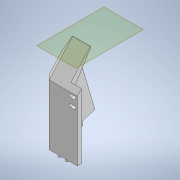
# Autodesk Inventor part: blotnik_v3_part_1
Saved by Autodesk Inventor 2022.3 (Build 263350000, 350)
## iProperties
Created: 2022-10-25
Part Number: blotnik_v3_part_1
Material: Generic
Document SubType Name: Modeling
Designer: Kamil
Density: 1 g/cm^3
Appearance: Default
Author: Kamil
Autodesk Inventor part; units mm, degrees
(part 1 of 2)
ref_plane "YZ Plane" through (0, 0, 0) normal (1, 0, 0) x (0, 1, 0)
ref_plane "XZ Plane" through (0, 0, 0) normal (0, 1, 0) x (-1, 0, 0)
sketch "Sketch1" plane through (0, 0, 0) normal (1, 0, 0) x (0, 1, 0)
  line L0 (-91.9132, 90.5719) -> (-91.9132, 0.5719)
  line L1 (-91.9132, 0.5719) -> (48.2351, 0.5719)
  arc A0 (48.2351, 0.5719) -> (67.9385, 0.5719) centre (58.0868, 2.2876) ccw
  line L2 (67.9385, 0.5719) -> (198.2351, 0.5719)
  arc A1 (198.2351, 0.5719) -> (217.9385, 0.5719) centre (208.0868, 2.2876) ccw
  line L3 (217.9385, 0.5719) -> (338.2351, 0.5719)
  arc A2 (338.2351, 0.5719) -> (357.9385, 0.5719) centre (348.0868, 2.2876) ccw
  line L4 (357.9385, 0.5719) -> (387.824, 0.5719)
  arc A3 (387.824, 0.5719) -> (392.824, 1.9116) centre (387.824, 10.5719) ccw
  line L5 (392.824, 1.9116) -> (465.5868, 43.9213)
  arc A4 (465.5868, 43.9213) -> (453.0868, 90.5719) centre (453.0868, 65.5719) ccw
  line L6 (453.0868, 90.5719) -> (215.5868, 90.5719)
  arc A5 (215.5868, 90.5719) -> (200.5868, 90.5719) centre (208.0868, 90.5719) ccw
  line L7 (200.5868, 90.5719) -> (65.5868, 90.5719)
  arc A6 (65.5868, 90.5719) -> (50.5868, 90.5719) centre (58.0868, 90.5719) ccw
  line L8 (50.5868, 90.5719) -> (-91.9132, 90.5719)
  line L9 (394.4234, 30.0809) -> (384.8369, 44.4607)
  arc A7 (384.8369, 46.6796) -> (384.8369, 44.4607) centre (386.501, 45.5701) ccw
  line L10 (384.8369, 46.6796) -> (394.4264, 61.0622)
  arc A8 (398.0904, 59.9525) -> (394.4264, 61.0622) centre (396.0904, 59.9527) ccw
  line L11 (398.0904, 59.9525) -> (398.0875, 31.1901)
  arc A9 (394.4234, 30.0809) -> (398.0875, 31.1901) centre (396.0875, 31.1903) ccw
  line L12 (46.0868, 47.6815) -> (11.9586, 47.6815)
  arc A10 (11.0641, 51.4704) -> (11.9586, 47.6815) centre (11.9586, 49.6815) ccw
  line L13 (11.0641, 51.4704) -> (45.1924, 68.5345)
  arc A11 (48.0868, 66.7457) -> (45.1924, 68.5345) centre (46.0868, 66.7457) ccw
  line L14 (48.0868, 66.7457) -> (48.0868, 49.6815)
  arc A12 (46.0868, 47.6815) -> (48.0868, 49.6815) centre (46.0868, 49.6815) ccw
  line L15 (278.9812, 39.5345) -> (319.3287, 19.3608)
  arc A13 (318.4343, 15.5719) -> (319.3287, 19.3608) centre (318.4343, 17.5719) ccw
  line L16 (318.4343, 15.5719) -> (237.7393, 15.5719)
  arc A14 (236.8448, 19.3608) -> (237.7393, 15.5719) centre (237.7393, 17.5719) ccw
  line L17 (236.8448, 19.3608) -> (277.1924, 39.5345)
  arc A15 (278.9812, 39.5345) -> (277.1924, 39.5345) centre (278.0868, 37.7457) ccw
  line L18 (367.8331, 75.5719) -> (388.3444, 75.5719)
  arc A16 (390.0084, 72.4624) -> (388.3444, 75.5719) centre (388.3444, 73.5719) ccw
  line L19 (390.0084, 72.4624) -> (379.7522, 57.0798)
  arc A17 (376.4241, 57.0798) -> (379.7522, 57.0798) centre (378.0882, 58.1892) ccw
  line L20 (376.4241, 57.0798) -> (366.169, 72.4625)
  arc A18 (367.8331, 75.5719) -> (366.169, 72.4625) centre (367.8331, 73.5719) ccw
  line L21 (361.7509, 61.0619) -> (371.3389, 46.6799)
  arc A19 (371.3388, 44.461) -> (371.3389, 46.6799) centre (369.6748, 45.5705) ccw
  line L22 (371.3388, 44.461) -> (361.7508, 30.0806)
  arc A20 (358.0868, 31.1901) -> (361.7508, 30.0806) centre (360.0868, 31.1901) ccw
  line L23 (358.0868, 31.1901) -> (358.0868, 59.9525)
  arc A21 (361.7509, 61.0619) -> (358.0868, 59.9525) centre (360.0868, 59.9525) ccw
  line L24 (89.1243, 75.5719) -> (177.0493, 75.5719)
  arc A22 (177.8875, 71.756) -> (177.0493, 75.5719) centre (177.0493, 73.5719) ccw
  line L25 (177.8875, 71.756) -> (133.9249, 51.4656)
  arc A23 (132.2487, 51.4656) -> (133.9249, 51.4656) centre (133.0868, 53.2815) ccw
  line L26 (132.2487, 51.4656) -> (88.2861, 71.756)
  arc A24 (89.1243, 75.5719) -> (88.2861, 71.756) centre (89.1243, 73.5719) ccw
  line L27 (-11.0188, 39.5345) -> (29.3287, 19.3608)
  arc A25 (28.4343, 15.5719) -> (29.3287, 19.3608) centre (28.4343, 17.5719) ccw
  line L28 (28.4343, 15.5719) -> (-52.2607, 15.5719)
  arc A26 (-53.1552, 19.3608) -> (-52.2607, 15.5719) centre (-52.2607, 17.5719) ccw
  line L29 (-53.1552, 19.3608) -> (-12.8076, 39.5345)
  arc A27 (-11.0188, 39.5345) -> (-12.8076, 39.5345) centre (-11.9132, 37.7457) ccw
  line L30 (117.2208, 43.756) -> (70.9249, 22.3887)
  arc A28 (68.0868, 24.2046) -> (70.9249, 22.3887) centre (70.0868, 24.2046) ccw
  line L31 (68.0868, 24.2046) -> (68.0868, 66.9392)
  arc A29 (70.9249, 68.7551) -> (68.0868, 66.9392) centre (70.0868, 66.9392) ccw
  line L32 (70.9249, 68.7551) -> (117.2208, 47.3878)
  arc A30 (117.2208, 43.756) -> (117.2208, 47.3878) centre (116.3827, 45.5719) ccw
  line L33 (-71.9132, 24.3981) -> (-71.9132, 66.7457)
  arc A31 (-69.0188, 68.5345) -> (-71.9132, 66.7457) centre (-69.9132, 66.7457) ccw
  line L34 (-69.0188, 68.5345) -> (-26.6713, 47.3608)
  arc A32 (-26.6713, 43.783) -> (-26.6713, 47.3608) centre (-27.5657, 45.5719) ccw
  line L35 (-26.6713, 43.783) -> (-69.0188, 22.6093)
  arc A33 (-71.9132, 24.3981) -> (-69.0188, 22.6093) centre (-69.9132, 24.3981) ccw
  line L36 (177.0493, 15.5719) -> (89.1243, 15.5719)
  arc A34 (88.2861, 19.3878) -> (89.1243, 15.5719) centre (89.1243, 17.5719) ccw
  line L37 (88.2861, 19.3878) -> (132.2487, 39.6782)
  arc A35 (133.9249, 39.6782) -> (132.2487, 39.6782) centre (133.0868, 37.8623) ccw
  line L38 (133.9249, 39.6782) -> (177.8875, 19.3878)
  arc A36 (177.0493, 15.5719) -> (177.8875, 19.3878) centre (177.0493, 17.5719) ccw
  line L39 (330.1924, 25.1093) -> (292.8448, 43.783)
  arc A37 (292.8448, 47.3608) -> (292.8448, 43.783) centre (293.7393, 45.5719) ccw
  line L40 (292.8448, 47.3608) -> (330.1924, 66.0345)
  arc A38 (333.0868, 64.2457) -> (330.1924, 66.0345) centre (331.0868, 64.2457) ccw
  line L41 (333.0868, 64.2457) -> (333.0868, 26.8981)
  arc A39 (330.1924, 25.1093) -> (333.0868, 26.8981) centre (331.0868, 26.8981) ccw
  line L42 (379.7517, 34.0607) -> (390.0046, 18.6813)
  arc A40 (388.3405, 15.5719) -> (390.0046, 18.6813) centre (388.3405, 17.5719) ccw
  line L43 (388.3405, 15.5719) -> (367.8335, 15.5719)
  arc A41 (366.1695, 18.6814) -> (367.8335, 15.5719) centre (367.8335, 17.5719) ccw
  line L44 (366.1695, 18.6814) -> (376.4235, 34.0608)
  arc A42 (379.7517, 34.0607) -> (376.4235, 34.0608) centre (378.0876, 32.9513) ccw
  line L45 (237.7393, 75.5719) -> (318.4343, 75.5719)
  arc A43 (319.3287, 71.783) -> (318.4343, 75.5719) centre (318.4343, 73.5719) ccw
  line L46 (319.3287, 71.783) -> (278.9812, 51.6093)
  arc A44 (277.1924, 51.6093) -> (278.9812, 51.6093) centre (278.0868, 53.3981) ccw
  line L47 (277.1924, 51.6093) -> (236.8448, 71.783)
  arc A45 (237.7393, 75.5719) -> (236.8448, 71.783) centre (237.7393, 73.5719) ccw
  line L48 (196.0868, 47.6815) -> (158.6952, 47.6815)
  arc A46 (157.857, 51.4975) -> (158.6952, 47.6815) centre (158.6952, 49.6815) ccw
  line L49 (157.857, 51.4975) -> (195.2487, 68.7551)
  arc A47 (198.0868, 66.9392) -> (195.2487, 68.7551) centre (196.0868, 66.9392) ccw
  line L50 (198.0868, 66.9392) -> (198.0868, 49.6815)
  arc A48 (196.0868, 47.6815) -> (198.0868, 49.6815) centre (196.0868, 49.6815) ccw
  line L51 (-52.2607, 75.5719) -> (28.4343, 75.5719)
  arc A49 (29.3287, 71.783) -> (28.4343, 75.5719) centre (28.4343, 73.5719) ccw
  line L52 (29.3287, 71.783) -> (-11.0188, 51.6093)
  arc A50 (-12.8076, 51.6093) -> (-11.0188, 51.6093) centre (-11.9132, 53.3981) ccw
  line L53 (-12.8076, 51.6093) -> (-53.1552, 71.783)
  arc A51 (-52.2607, 75.5719) -> (-53.1552, 71.783) centre (-52.2607, 73.5719) ccw
  line L54 (220.9812, 68.5345) -> (263.3287, 47.3608)
  arc A52 (263.3287, 43.783) -> (263.3287, 47.3608) centre (262.4343, 45.5719) ccw
  line L55 (263.3287, 43.783) -> (220.9812, 22.6093)
  arc A53 (218.0868, 24.3981) -> (220.9812, 22.6093) centre (220.0868, 24.3981) ccw
  line L56 (218.0868, 24.3981) -> (218.0868, 66.7457)
  arc A54 (220.9812, 68.5345) -> (218.0868, 66.7457) centre (220.0868, 66.7457) ccw
  circle A55 centre (208.0868, 2.2876) radius 2.5
  circle A56 centre (348.0868, 2.2876) radius 2.5
  circle A57 centre (243.0868, 8.0719) radius 2.5
  circle A58 centre (183.0868, 37.6815) radius 2.5
  circle A59 centre (23.0868, 37.6815) radius 2.5
  circle A60 centre (-81.9132, 83.0719) radius 2.5
  circle A61 centre (100.0868, 83.0715) radius 2.5
  circle A62 centre (260.0868, 83.0715) radius 2.5
  circle A63 centre (343.0868, 37.6815) radius 2.5
  circle A64 centre (348.0868, 83.0719) radius 2.5
  circle A65 centre (58.0868, 2.2876) radius 2.5
  circle A66 centre (-81.9132, 8.0719) radius 2.5
  line L57 (413.0868, 68.5719) -> (453.0868, 68.5719)
  arc A67 (453.0868, 62.5719) -> (453.0868, 68.5719) centre (453.0868, 65.5719) ccw
  line L58 (453.0868, 62.5719) -> (413.0868, 62.5719)
  arc A68 (413.0868, 68.5719) -> (413.0868, 62.5719) centre (413.0868, 65.5719) ccw
  line L59 (493.0868, 110.5719) -> (493.0868, -89.4281)
  line L60 (493.0868, -89.4281) -> (-191.9132, -89.4281)
  circle A69 centre (453.0868, 65.5719) radius 40
  circle A70 centre (-151.9132, 65.5719) radius 40
  line L61 (493.0868, -89.4281) -> (-191.9132, -89.4281)
  line L62 (-191.9132, -89.4281) -> (-191.9132, -23.4281)
  line L63 (-191.9132, -23.4281) -> (493.0868, -23.4281)
  line L64 (493.0868, -23.4281) -> (493.0868, -89.4281)
  line L65 (493.0868, -89.4281) -> (513.0868, -89.4281)
  line L66 (493.0868, 111.0798) -> (493.0868, -89.4281)
  line L67 (453.0868, 65.5719) -> (503.1002, 121.4616)
  line L68 (479.7606, 95.3797) -> (493.0975, 110.2837)
  line L69 (493.0975, 110.2837) -> (453.6631, 145.5719)
  line L70 (453.6631, 145.5719) -> (531.8877, 75.5719)
  line L71 (-151.9132, 65.5719) -> (-191.775, 110.4165)
  line L72 (-178.4878, 95.4683) -> (-191.775, 110.4165)
  line L73 (-191.775, 110.4165) -> (-234.9459, 72.0424)
  line L74 (-234.9459, 72.0424) -> (-158.1796, 140.2791)
  line L75 (528.0086, -89.3576) -> (513.0086, -89.3576)
  line L76 (518.0059, 87.9942) -> (528.0086, 99.1721)
  line L77 (465.5868, 134.9019) -> (475.5895, 146.0798)
  line L78 (532.1476, 95.4683) -> (475.5895, 146.0798)
  line L79 (475.5895, 146.0798) -> (554.3817, 75.5719)
  line L80 (518.0059, 87.9942) -> (531.8877, 75.5719)
  line L81 (543.0627, 75.5719) -> (584.6456, 75.5719)
  line L82 (584.6456, 75.5719) -> (398.3496, 75.5719)
  line L83 (-158.1796, 140.2791) -> (-132.7437, 162.756)
  line L84 (-226.9914, -89.3576) -> (-211.9914, -89.3576)
  line L85 (-250.1298, 130.5719) -> (-250.1298, 145.5719)
  line L86 (-191.9132, -89.4281) -> (-191.9132, 65.5719)
  line L87 (-191.9132, 110.2936) -> (-191.9132, 110.5719)
  line L88 (-191.9132, 110.2936) -> (-201.8787, 121.5048)
  line L89 (-201.8885, 121.496) -> (-174.8032, 145.5719)
  line L90 (-201.8885, 121.496) -> (-254.6566, 74.591)
  line L91 (-211.9132, -4.094) -> (-211.9132, 29.4476)
  line L92 (-191.9132, 29.4476) -> (-191.9132, -4.094)
  line L93 (-226.9132, -4.094) -> (-226.9132, 29.4476)
  line L94 (-211.9132, 29.4476) -> (-211.9132, -4.094)
  line L95 (-226.9132, -4.094) -> (-211.9132, -4.094)
  line L96 (-211.9132, -4.094) -> (-211.9132, 115.8992)
  line L97 (-211.9132, 115.8992) -> (-226.9132, 115.8992)
  line L98 (-226.9132, 115.8992) -> (-226.9132, -4.094)
  line L99 (-226.9132, -4.094) -> (-211.9132, -4.094)
  line L100 (-211.9132, -4.094) -> (-211.9132, -158.3275)
  line L101 (-211.9132, -158.3275) -> (-226.9132, -158.3275)
  line L102 (-226.9132, -158.3275) -> (-226.9132, -4.094)
  line L103 (531.8877, 75.5719) -> (543.891, 88.9854)
  line L104 (-191.9132, 110.2936) -> (-203.8718, 123.747)
  line L105 (-211.9132, -4.094) -> (-229.9132, -4.094)
  line L106 (-229.9132, -4.094) -> (-229.9132, 127.9278)
  line L107 (-229.9132, 127.9278) -> (-229.9132, -180.4745)
  line L108 (-203.8718, 123.747) -> (-168.2156, 155.4414)
  line L109 (-168.2156, 155.4414) -> (-240.454, 91.2294)
  line L110 (543.891, 88.9854) -> (459.9065, 164.1396)
  line L111 (459.9065, 164.1396) -> (563.8541, 71.1212)
  circle A71 centre (348.0868, 83.0719) radius 6.7103
  circle A72 centre (-81.9132, 8.0719) radius 5.7664
  line L112 (-211.9132, -23.4281) -> (-229.9132, -23.4281)
  line L113 (493.0868, -23.4281) -> (732.785, -23.4281)
  line L114 (558.8805, 75.5719) -> (222.3331, -23.4281)
  line L115 (222.3331, -23.4281) -> (-229.9132, -23.4281)
  line L116 (453.0868, 105.5719) -> (495.4894, 105.5719)
  line L117 (453.0868, 105.5719) -> (453.0868, 123.5719)
  line L118 (453.0868, 123.5719) -> (517.1971, 123.5719)
  line L119 (453.0868, 123.5719) -> (453.0868, 138.5719)
  line L120 (453.0868, 138.5719) -> (512.6454, 138.5719)
  line L121 (453.0868, 138.5719) -> (-211.9132, 138.5719)
  line L122 (453.0868, 123.5719) -> (-280.7499, 123.5719)
  point P0 (0, 0)
  point P1 (0, 0)
  point P2 (558.8805, 75.5719)
  point P3 (488.4783, 138.5719)
  point P4 (-187.1938, 138.5719)
  point P5 (-203.7161, 123.5719)
  point P6 (-204.0688, 123.5719)
  point P7 (-229.9132, 100.599)
  point P8 (-211.9132, 92.5159)
  point P9 (-176.9752, 123.5719)
  point P10 (478.248, 123.5719)
  point P11 (493.0868, 110.2933)
  point P12 (493.0868, 110.2717)
  dimension "d2" = 685
  dimension "d3" = 200
  dimension "d9" = 20
  dimension "d11" = 20
  dimension "d13" = 15
  dimension "d14" = 15
  dimension "d15" = 15
  dimension "d20" = 15
  dimension "d23" = 18
  dimension "d25" = 18
  dimension "d26" = 18
  dimension "d28" = 18
  dimension "d29" = 15
  constraints: 246 end point, 118 point on circle, 73 centre point, 26 point on line, 17 perpendicular, 12 parallel, 7 horizontal, 3 coincident, 3 tangent, 2 vertical, 1 collinear
  measures "d2" distance of L59.start L87.end
  measures "d3" distance of L59.start L59.end
  measures "d9" distance of L68.start L68.end
  measures "d11" distance of L71.end L72.start
  measures "d13" distance of L75.start L75.end
  measures "d14" distance of L76.start L76.end
  measures "d15" distance of L77.end L77.start
  measures "d20" distance of L87.start L88.end
  measures "d23" distance of L70.end L103.end
  measures "d25" distance of L87.start L104.end
  measures "d26" distance of L99.end L105.end
  measures "d28" distance of L116.start L117.end
  measures "d29" distance of L117.end L119.end
extrude "Extrusion1" add sketch "Sketch1" along normal blind 100 contours L119 L120 L69 L118 | L122 L74 L121 L119 | L118 L78 L67 L69 | L69 L77 L120 L78 L118 | L122 L89 L121 L74 | L74 L73 L88 L89 L122 | L112 L102 L95 L100 | L67 L78 L76 L70 | L69 L120 L77 | L118 L110 L103 L79 L78 | L78 L120 L110 L118 | L122 L104 L108 L121 L89 | L89 L104 L122 | L95 L93 L98 L73 L96 L91 | L112 L107 L105 L102 | L81 L79 L103 L111 | L103 L79 L81 L82 | L70 L76 L78 L79 L103 | L73 L96 L90 L89 L88 | L89 L90 L96 L97 L109 L122 L104 | L105 L106 L73 L98 L93 | L73 L98 L90 L96 | L73 L106 L90 L98 | L90 L98 L109 L97 L96 | L90 L106 L109 L98
extrude "Extrusion2" add sketch "Sketch1" against normal blind 20 contours L8 A6 L7 A5 L6 A69 L57 A68 L58 L114 L42 A42 L44 L3 A1 L2 A0 L1 L0 | L0 L1 A0 L2 A1 L3 L114 L63 L86 A70 L71 L74 L122 L117 A69 L6 A5 L7 A6 L8 | A69 L67 A4 L6 | L6 A4 L67 L82 A69 | L116 L67 A69 | L117 L118 L69 L59 L67 L116 | L82 L67 A67 L57 A69 | L44 A42 L42 L114 | L67 A69 L82 A4 | A4 L82 L67 | L67 L116 L59 L82 A69 | L67 L59 L116 | L119 L120 L69 L118 | L122 L74 L121 L119 | A69 L58 A68 L57 | L57 A67 L58 A69 | L82 A4 L114 A69 L58 A67 L67 | L115 L100 L91 L96 L73 L71 A70 L86 | L82 A69 L114 A4 | L82 L59 A69 | L67 L70 L82 L59 | L118 L78 L67 L69 | L69 L77 L120 L78 L118 | L122 L89 L121 L74 | L74 L73 L88 L89 L122 | L112 L102 L95 L100 | L114 A69 L59 | L59 L82 L81 L114 | L67 L78 L76 L70 | L69 L120 L77 | L118 L110 L103 L79 L78 | L78 L120 L110 L118 | L122 L104 L108 L121 L89 | L89 L104 L122 | L95 L93 L98 L73 L96 L91 | L112 L107 L105 L102 | L81 L79 L103 L111 | L103 L79 L81 L82 | L70 L76 L78 L79 L103 | A70 | L73 L96 L90 L89 L88 | L89 L90 L96 L97 L109 L122 L104 | L122 L109 L104 | L105 L106 L73 L98 L93 | L73 L98 L90 L96 | L73 L106 L90 L98 | L90 L98 L109 L97 L96 | L90 L106 L109 L98 | L9 A7 L10 A8 L11 A9 | L12 A10 L13 A11 L14 A12 | L15 A13 L16 A14 L17 A15 | L18 A16 L19 A17 L20 A18 | L21 A19 L22 A20 L23 A21 | L24 A22 L25 A23 L26 A24 | L27 A25 L28 A26 L29 A27 | L30 A28 L31 A29 L32 A30 | L33 A31 L34 A32 L35 A33 | L36 A34 L37 A35 L38 A36 | L39 A37 L40 A38 L41 A39 | L45 A43 L46 A44 L47 A45 | L48 A46 L49 A47 L50 A48 | L51 A49 L52 A50 L53 A51 | L54 A52 L55 A53 L56 A54 | A55 | A57 | A58 | A59 | A60 | A61 | A62 | A63 | A65
chamfer "Chamfer1" distance 20 angle 45 6 edges at (-20, 523.6794, 107.0719) (-20, 390.6068, 26.0719) (-20, -3.7901, -23.4281) (-20, 150.6423, 138.5719) (-20, -208.5535, 119.5855) (-20, -229.9132, 38.5855)
sketch "Sketch2" plane through (100, 0, 0) normal (1, 0, 0) x (0, 0, -1)
  line L0 (-123.5719, 478.248) -> (-75.5719, 531.8877) projected
  line L1 (-75.5719, 531.8877) -> (-75.5719, 558.8805) projected
  line L2 (-75.5719, 558.8805) -> (-138.5719, 488.4783) projected
  line L3 (-138.5719, 488.4783) -> (-138.5719, -187.1938) projected
  line L4 (-138.5719, -187.1938) -> (-123.747, -203.8718) projected
  line L5 (-123.747, -203.8718) -> (-123.5719, -203.7161) projected
  line L6 (-123.5719, -203.7161) -> (-123.5719, -204.0688) projected
  line L7 (-123.5719, -204.0688) -> (-100.599, -229.9132) projected
  line L8 (-100.599, -229.9132) -> (23.4281, -229.9132) projected
  line L9 (23.4281, -229.9132) -> (23.4281, -211.9132) projected
  line L10 (23.4281, -211.9132) -> (-92.5159, -211.9132) projected
  line L11 (-92.5159, -211.9132) -> (-123.5719, -176.9752) projected
  line L12 (-123.5719, -176.9752) -> (-123.5719, 478.248) projected
  line L13 (-123.5719, -203.7161) -> (-123.5719, -204.0688) projected
  line L14 (-123.747, -203.8718) -> (-123.5719, -204.0688)
  point P0 (0, 0)
  constraints: 2 end point
extrude "Extrusion3" add sketch "Sketch2" against normal up to surface (100 mm away) contours L5 L6 L14
sketch "Sketch3" plane through (100, -187.1938, 138.5719) normal (0, 0, 1) x (1, 0, 0)
  line L0 (-100, 0) -> (-100, 675.6721) projected
  line L1 (-100, 0) -> (0, 0) projected
  line L2 (0, 675.6721) -> (0, 0) projected
  line L3 (-100, 675.6721) -> (0, 675.6721) projected
  line L4 (-100, 0) -> (-25, 0)
  line L5 (-25, 0) -> (-25, 62.1275)
  line L6 (-25, 62.1275) -> (-100, 62.1275)
  line L7 (-100, 62.1275) -> (-100, 0)
  line L8 (-100, -42.7195) -> (0, -42.7195) projected
  line L9 (-25, -42.7195) -> (80.9941, -42.7195)
  line L10 (80.9941, -42.7195) -> (80.9941, 814.1524)
  line L11 (80.9941, 814.1524) -> (-25, 814.1524)
  line L12 (-25, 814.1524) -> (-25, -42.7195)
  point P0 (-100, 187.1938)
  dimension "d45" = 75
  constraints: 16 end point, 4 parallel, 2 horizontal, 2 perpendicular, 2 point on line
  measures "d45" distance of L6.end L5.end
extrude "Extrusion4" cut sketch "Sketch3" against normal through all contours L5 L12 L3 L2 L1 | L1 L2 L3 L12 L11 L10 L9 L8
sketch "Sketch4" plane through (0, 0, 0) normal (1, 0, 0) x (0, 0, -1)
  line L0 (23.4281, -211.9132) -> (23.4281, 222.3331) projected
  line L1 (23.4281, 222.3331) -> (-75.5719, 558.8805) projected
  line L2 (-75.5719, 531.8877) -> (-75.5719, 558.8805) projected
  circle A0 centre (-8.0719, -81.9132) radius 5.7664 projected
  circle A1 centre (-83.0719, 348.0868) radius 6.7103 projected
  circle A2 centre (-8.0719, -81.9132) radius 11.2282
  circle A3 centre (-83.0719, 348.0868) radius 6.7103 projected
  circle A4 centre (-83.0719, 348.0868) radius 15.3296
  line L3 (-123.5719, -176.9752) -> (-123.5719, 478.248) projected
  line L4 (-92.5159, -211.9132) -> (-123.5719, -176.9752) projected
  line L5 (23.4281, -211.9132) -> (-92.5159, -211.9132) projected
  line L6 (-110.2837, 493.0975) -> (-75.5719, 531.8877) projected
  line L7 (-110.2837, 493.0975) -> (-110.2717, 493.0868) projected
  line L8 (-110.2717, 493.0868) -> (-110.2933, 493.0868) projected
  line L9 (-123.5719, 478.248) -> (-110.2933, 493.0868) projected
  point P0 (0, 0)
  constraints: 2 centre point, 2 coincident
extrude "Extrusion5" add sketch "Sketch4" along normal blind 15 contours A2 | A4
sketch "Sketch5" plane through (0, -187.1938, 138.5719) normal (0, 0, 1) x (1, 0, 0)
  line L0 (75, 0) -> (75, 675.6721) projected
  line L1 (0, 675.6721) -> (75, 675.6721) projected
  line L2 (0, 0) -> (0, 675.6721) projected
  line L3 (0, 0) -> (75, 0) projected
  line L4 (10, 71.8086) -> (65, 71.8086)
  line L5 (65, 71.8086) -> (65, 16)
  line L6 (65, 16) -> (10, 16)
  line L7 (10, 16) -> (10, 71.8086)
  line L8 (75, 665.4417) -> (75, 10.2186) projected
  line L9 (0, 0) -> (75, 0)
  line L10 (75, 0) -> (75, 16)
  line L11 (75, 16) -> (0, 16)
  line L12 (0, 16) -> (0, 0)
  line L13 (75, 337.8302) -> (0, 337.8245)
  line L14 (0, 12.4998) -> (0, 663.1491) projected
  line L15 (10, 71.8086) -> (65, 71.8086)
  line L16 (65, 71.8086) -> (65, 325.2511)
  line L17 (65, 325.2511) -> (10, 325.2511)
  line L18 (10, 325.2511) -> (10, 71.8086)
  line L19 (0, 675.6721) -> (75, 675.6721)
  line L20 (75, 675.6721) -> (75, 659.6721)
  line L21 (75, 659.6721) -> (0, 659.6721)
  line L22 (0, 659.6721) -> (0, 675.6721)
  line L23 (10, 325.2511) -> (65, 325.2511)
  line L24 (65, 325.2511) -> (65, 659.6721)
  line L25 (65, 659.6721) -> (10, 659.6721)
  line L26 (10, 659.6721) -> (10, 325.2511)
  line L27 (10, 348.6782) -> (10, 311.2591)
  point P0 (0, 187.1938)
  point P1 (37.5, 16)
  point P2 (37.5, 16)
  point P3 (10, 325.2511)
  point P4 (65, 71.8086)
  point P5 (10, 659.6721)
  dimension "d50" = 55
  dimension "d51" = 16
  dimension "d52" = 16
  constraints: 44 end point, 10 parallel, 5 horizontal, 5 perpendicular, 5 point on line, 4 midpoint
  measures "d50" distance of L5.end L6.end
  measures "d51" distance of L10.end L9.end
  measures "d52" distance of L19.end L20.end
extrude "Extrusion6" cut sketch "Sketch5" against normal blind 4 contours L6 L7 L4 L5 | L24 L17 L26 L13 | L13 L26 L21 L24 | L4 L18 L17 L16
sketch "Sketch6" plane through (0, 0, 0) normal (1, 0, 0) x (0, 0, -1)
  circle A0 centre (-83.0719, -81.9132) radius 2.5 projected
  circle A1 centre (-83.0719, -81.9132) radius 9.5792
  circle A2 centre (-83.0719, -81.9132) radius 3.9821
  point P0 (0, 0)
  constraints: 2 centre point, 2 coincident
extrude "Extrusion7" add sketch "Sketch6" along normal up to surface (15 mm away) contours A1
sketch "Sketch7" plane through (0, 0, 0) normal (1, 0, 0) x (0, 0, -1)
  circle A0 centre (-37.6815, 343.0868) radius 2.5 projected
  circle A1 centre (-37.6815, 343.0868) radius 3
  circle A2 centre (-37.6815, 343.0868) radius 7.0135
  point P0 (0, 0)
  dimension "d57" = 6
  constraints: 2 centre point, 2 coincident
  measures "d57" diameter of A1
extrude "Extrusion8" add sketch "Sketch7" along normal up to surface (15 mm away) contours A2
sketch "Sketch9" plane through (-20, 0, 0) normal (-1, 0, 0) x (0, 0, 1)
  line L0 (90.5719, -91.9132) -> (0.5719, -91.9132) projected
  line L1 (0.5719, -91.9132) -> (0.5719, 48.2351) projected
  arc A0 (0.5719, 67.9385) -> (0.5719, 48.2351) centre (2.2876, 58.0868) ccw projected
  line L2 (0.5719, 67.9385) -> (0.5719, 198.2351) projected
  arc A1 (0.5719, 217.9385) -> (0.5719, 198.2351) centre (2.2876, 208.0868) ccw projected
  line L3 (0.5719, 217.9385) -> (0.5719, 338.2351) projected
  arc A2 (0.5719, 357.9385) -> (0.5719, 338.2351) centre (2.2876, 348.0868) ccw projected
  line L4 (0.5719, 357.9385) -> (0.5719, 387.824) projected
  arc A3 (1.9116, 392.824) -> (0.5719, 387.824) centre (10.5719, 387.824) ccw projected
  line L5 (1.9116, 392.824) -> (43.9213, 465.5868) projected
  arc A4 (90.5719, 453.0868) -> (43.9213, 465.5868) centre (65.5719, 453.0868) ccw projected
  line L6 (90.5719, 453.0868) -> (90.5719, 215.5868) projected
  arc A5 (90.5719, 200.5868) -> (90.5719, 215.5868) centre (90.5719, 208.0868) ccw projected
  line L7 (90.5719, 200.5868) -> (90.5719, 65.5868) projected
  arc A6 (90.5719, 50.5868) -> (90.5719, 65.5868) centre (90.5719, 58.0868) ccw projected
  line L8 (90.5719, 50.5868) -> (90.5719, -91.9132) projected
  line L9 (30.0809, 394.4234) -> (44.4607, 384.8369) projected
  arc A7 (44.4607, 384.8369) -> (46.6796, 384.8369) centre (45.5701, 386.501) ccw projected
  line L10 (46.6796, 384.8369) -> (61.0622, 394.4264) projected
  arc A8 (61.0622, 394.4264) -> (59.9525, 398.0904) centre (59.9527, 396.0904) ccw projected
  line L11 (59.9525, 398.0904) -> (31.1901, 398.0875) projected
  arc A9 (31.1901, 398.0875) -> (30.0809, 394.4234) centre (31.1903, 396.0875) ccw projected
  line L12 (47.6815, 46.0868) -> (47.6815, 11.9586) projected
  arc A10 (47.6815, 11.9586) -> (51.4704, 11.0641) centre (49.6815, 11.9586) ccw projected
  line L13 (51.4704, 11.0641) -> (68.5345, 45.1924) projected
  arc A11 (68.5345, 45.1924) -> (66.7457, 48.0868) centre (66.7457, 46.0868) ccw projected
  line L14 (66.7457, 48.0868) -> (49.6815, 48.0868) projected
  arc A12 (49.6815, 48.0868) -> (47.6815, 46.0868) centre (49.6815, 46.0868) ccw projected
  line L15 (39.5345, 278.9812) -> (19.3608, 319.3287) projected
  arc A13 (19.3608, 319.3287) -> (15.5719, 318.4343) centre (17.5719, 318.4343) ccw projected
  line L16 (15.5719, 318.4343) -> (15.5719, 237.7393) projected
  arc A14 (15.5719, 237.7393) -> (19.3608, 236.8448) centre (17.5719, 237.7393) ccw projected
  line L17 (19.3608, 236.8448) -> (39.5345, 277.1924) projected
  arc A15 (39.5345, 277.1924) -> (39.5345, 278.9812) centre (37.7457, 278.0868) ccw projected
  line L18 (75.5719, 367.8331) -> (75.5719, 388.3444) projected
  arc A16 (75.5719, 388.3444) -> (72.4624, 390.0084) centre (73.5719, 388.3444) ccw projected
  line L19 (72.4624, 390.0084) -> (57.0798, 379.7522) projected
  arc A17 (57.0798, 379.7522) -> (57.0798, 376.4241) centre (58.1892, 378.0882) ccw projected
  line L20 (57.0798, 376.4241) -> (72.4625, 366.169) projected
  arc A18 (72.4625, 366.169) -> (75.5719, 367.8331) centre (73.5719, 367.8331) ccw projected
  line L21 (61.0619, 361.7509) -> (46.6799, 371.3389) projected
  arc A19 (46.6799, 371.3389) -> (44.461, 371.3388) centre (45.5705, 369.6748) ccw projected
  line L22 (44.461, 371.3388) -> (30.0806, 361.7508) projected
  arc A20 (30.0806, 361.7508) -> (31.1901, 358.0868) centre (31.1901, 360.0868) ccw projected
  line L23 (31.1901, 358.0868) -> (59.9525, 358.0868) projected
  arc A21 (59.9525, 358.0868) -> (61.0619, 361.7509) centre (59.9525, 360.0868) ccw projected
  line L24 (75.5719, 89.1243) -> (75.5719, 177.0493) projected
  arc A22 (75.5719, 177.0493) -> (71.756, 177.8875) centre (73.5719, 177.0493) ccw projected
  line L25 (71.756, 177.8875) -> (51.4656, 133.9249) projected
  arc A23 (51.4656, 133.9249) -> (51.4656, 132.2487) centre (53.2815, 133.0868) ccw projected
  line L26 (51.4656, 132.2487) -> (71.756, 88.2861) projected
  arc A24 (71.756, 88.2861) -> (75.5719, 89.1243) centre (73.5719, 89.1243) ccw projected
  line L27 (39.5345, -11.0188) -> (19.3608, 29.3287) projected
  arc A25 (19.3608, 29.3287) -> (15.5719, 28.4343) centre (17.5719, 28.4343) ccw projected
  line L28 (15.5719, 28.4343) -> (15.5719, -52.2607) projected
  arc A26 (15.5719, -52.2607) -> (19.3608, -53.1552) centre (17.5719, -52.2607) ccw projected
  line L29 (19.3608, -53.1552) -> (39.5345, -12.8076) projected
  arc A27 (39.5345, -12.8076) -> (39.5345, -11.0188) centre (37.7457, -11.9132) ccw projected
  line L30 (43.756, 117.2208) -> (22.3887, 70.9249) projected
  arc A28 (22.3887, 70.9249) -> (24.2046, 68.0868) centre (24.2046, 70.0868) ccw projected
  line L31 (24.2046, 68.0868) -> (66.9392, 68.0868) projected
  arc A29 (66.9392, 68.0868) -> (68.7551, 70.9249) centre (66.9392, 70.0868) ccw projected
  line L32 (68.7551, 70.9249) -> (47.3878, 117.2208) projected
  arc A30 (47.3878, 117.2208) -> (43.756, 117.2208) centre (45.5719, 116.3827) ccw projected
  line L33 (24.3981, -71.9132) -> (66.7457, -71.9132) projected
  arc A31 (66.7457, -71.9132) -> (68.5345, -69.0188) centre (66.7457, -69.9132) ccw projected
  line L34 (68.5345, -69.0188) -> (47.3608, -26.6713) projected
  arc A32 (47.3608, -26.6713) -> (43.783, -26.6713) centre (45.5719, -27.5657) ccw projected
  line L35 (43.783, -26.6713) -> (22.6093, -69.0188) projected
  arc A33 (22.6093, -69.0188) -> (24.3981, -71.9132) centre (24.3981, -69.9132) ccw projected
  line L36 (15.5719, 177.0493) -> (15.5719, 89.1243) projected
  arc A34 (15.5719, 89.1243) -> (19.3878, 88.2861) centre (17.5719, 89.1243) ccw projected
  line L37 (19.3878, 88.2861) -> (39.6782, 132.2487) projected
  arc A35 (39.6782, 132.2487) -> (39.6782, 133.9249) centre (37.8623, 133.0868) ccw projected
  line L38 (39.6782, 133.9249) -> (19.3878, 177.8875) projected
  arc A36 (19.3878, 177.8875) -> (15.5719, 177.0493) centre (17.5719, 177.0493) ccw projected
  line L39 (25.1093, 330.1924) -> (43.783, 292.8448) projected
  arc A37 (43.783, 292.8448) -> (47.3608, 292.8448) centre (45.5719, 293.7393) ccw projected
  line L40 (47.3608, 292.8448) -> (66.0345, 330.1924) projected
  arc A38 (66.0345, 330.1924) -> (64.2457, 333.0868) centre (64.2457, 331.0868) ccw projected
  line L41 (64.2457, 333.0868) -> (26.8981, 333.0868) projected
  arc A39 (26.8981, 333.0868) -> (25.1093, 330.1924) centre (26.8981, 331.0868) ccw projected
  line L42 (34.0607, 379.7517) -> (18.6813, 390.0046) projected
  arc A40 (18.6813, 390.0046) -> (15.5719, 388.3405) centre (17.5719, 388.3405) ccw projected
  line L43 (15.5719, 388.3405) -> (15.5719, 367.8335) projected
  arc A41 (15.5719, 367.8335) -> (18.6814, 366.1695) centre (17.5719, 367.8335) ccw projected
  line L44 (18.6814, 366.1695) -> (34.0608, 376.4235) projected
  arc A42 (34.0608, 376.4235) -> (34.0607, 379.7517) centre (32.9513, 378.0876) ccw projected
  line L45 (75.5719, 237.7393) -> (75.5719, 318.4343) projected
  arc A43 (75.5719, 318.4343) -> (71.783, 319.3287) centre (73.5719, 318.4343) ccw projected
  line L46 (71.783, 319.3287) -> (51.6093, 278.9812) projected
  arc A44 (51.6093, 278.9812) -> (51.6093, 277.1924) centre (53.3981, 278.0868) ccw projected
  line L47 (51.6093, 277.1924) -> (71.783, 236.8448) projected
  arc A45 (71.783, 236.8448) -> (75.5719, 237.7393) centre (73.5719, 237.7393) ccw projected
  line L48 (47.6815, 196.0868) -> (47.6815, 158.6952) projected
  arc A46 (47.6815, 158.6952) -> (51.4975, 157.857) centre (49.6815, 158.6952) ccw projected
  line L49 (51.4975, 157.857) -> (68.7551, 195.2487) projected
  arc A47 (68.7551, 195.2487) -> (66.9392, 198.0868) centre (66.9392, 196.0868) ccw projected
  line L50 (66.9392, 198.0868) -> (49.6815, 198.0868) projected
  arc A48 (49.6815, 198.0868) -> (47.6815, 196.0868) centre (49.6815, 196.0868) ccw projected
  line L51 (75.5719, -52.2607) -> (75.5719, 28.4343) projected
  arc A49 (75.5719, 28.4343) -> (71.783, 29.3287) centre (73.5719, 28.4343) ccw projected
  line L52 (71.783, 29.3287) -> (51.6093, -11.0188) projected
  arc A50 (51.6093, -11.0188) -> (51.6093, -12.8076) centre (53.3981, -11.9132) ccw projected
  line L53 (51.6093, -12.8076) -> (71.783, -53.1552) projected
  arc A51 (71.783, -53.1552) -> (75.5719, -52.2607) centre (73.5719, -52.2607) ccw projected
  line L54 (68.5345, 220.9812) -> (47.3608, 263.3287) projected
  arc A52 (47.3608, 263.3287) -> (43.783, 263.3287) centre (45.5719, 262.4343) ccw projected
  line L55 (43.783, 263.3287) -> (22.6093, 220.9812) projected
  arc A53 (22.6093, 220.9812) -> (24.3981, 218.0868) centre (24.3981, 220.0868) ccw projected
  line L56 (24.3981, 218.0868) -> (66.7457, 218.0868) projected
  arc A54 (66.7457, 218.0868) -> (68.5345, 220.9812) centre (66.7457, 220.0868) ccw projected
  circle A55 centre (2.2876, 208.0868) radius 2.5 projected
  circle A56 centre (2.2876, 348.0868) radius 2.5 projected
  circle A57 centre (8.0719, 243.0868) radius 2.5 projected
  circle A58 centre (37.6815, 183.0868) radius 2.5 projected
  circle A59 centre (37.6815, 23.0868) radius 2.5 projected
  circle A60 centre (83.0719, -81.9132) radius 2.5 projected
  circle A61 centre (83.0715, 100.0868) radius 2.5 projected
  circle A62 centre (83.0715, 260.0868) radius 2.5 projected
  circle A63 centre (37.6815, 343.0868) radius 2.5 projected
  circle A64 centre (83.0719, 348.0868) radius 2.5 projected
  circle A65 centre (2.2876, 58.0868) radius 2.5 projected
  circle A66 centre (8.0719, -81.9132) radius 2.5 projected
  line L57 (68.5719, 413.0868) -> (68.5719, 453.0868) projected
  arc A67 (68.5719, 453.0868) -> (62.5719, 453.0868) centre (65.5719, 453.0868) ccw projected
  line L58 (62.5719, 453.0868) -> (62.5719, 413.0868) projected
  arc A68 (62.5719, 413.0868) -> (68.5719, 413.0868) centre (65.5719, 413.0868) ccw projected
  circle A69 centre (37.6815, 343.0868) radius 3 projected
  circle A70 centre (37.6815, 343.0868) radius 3
  circle A71 centre (83.0715, 260.0868) radius 3
  circle A72 centre (37.6815, 183.0868) radius 3
  circle A73 centre (2.2876, 208.0868) radius 3
  circle A74 centre (2.2876, 58.0868) radius 3
  circle A75 centre (83.0715, 100.0868) radius 3
  circle A76 centre (83.0719, -81.9132) radius 3.9821 projected
  circle A77 centre (83.0719, -81.9132) radius 3.9821
  circle A78 centre (37.6815, 23.0868) radius 3
  point P0 (0, 0)
  dimension "d60" = 6
  dimension "d61" = 6
  dimension "d62" = 6
  dimension "d63" = 6
  dimension "d64" = 6
  dimension "d65" = 6
  constraints: 8 centre point, 8 coincident
  measures "d60" diameter of A71
  measures "d61" diameter of A72
  measures "d62" diameter of A73
  measures "d63" diameter of A74
  measures "d64" diameter of A75
  measures "d65" diameter of A78
extrude "Extrusion9" cut sketch "Sketch9" against normal through all contours A55 | A57 | A58 | A59 | A60 | A61 | A62 | A63 | A65 | A66 | A69 | A71 | A72 | A73 | A74 | A75 | A76 | A78
sketch "Sketch10" plane through (0, 0, 0) normal (1, 0, 0) x (0, 0, -1)
  circle A0 centre (-8.0719, 243.0868) radius 2.5 projected
  circle A1 centre (-2.2876, 58.0868) radius 3 projected
  circle A2 centre (-83.0715, 100.0868) radius 3 projected
  circle A3 centre (-83.0715, 260.0868) radius 3 projected
  circle A4 centre (-2.2876, 208.0868) radius 3 projected
  circle A5 centre (-37.6815, 23.0868) radius 3 projected
  circle A6 centre (-37.6815, 183.0868) radius 3 projected
  circle A7 centre (-83.0719, -81.9132) radius 9.5792 projected
  circle A8 centre (-83.0719, 348.0868) radius 15.3296 projected
  circle A9 centre (-8.0719, -81.9132) radius 11.2282 projected
  line L0 (23.4281, -211.9132) -> (23.4281, 222.3331) projected
  line L1 (23.4281, 222.3331) -> (-75.5719, 558.8805) projected
  line L2 (-75.5719, 531.8877) -> (-75.5719, 558.8805) projected
  circle A10 centre (-37.6815, 343.0868) radius 7.0135 projected
  circle A11 centre (-37.6815, 23.0868) radius 3 projected
  circle A12 centre (-37.6815, 23.0868) radius 10
  circle A13 centre (-83.0715, 100.0868) radius 3 projected
  circle A14 centre (-83.0715, 100.0868) radius 10
  circle A15 centre (-2.2876, 58.0868) radius 3 projected
  circle A16 centre (-2.2876, 58.0868) radius 10
  circle A17 centre (-37.6815, 183.0868) radius 3 projected
  circle A18 centre (-37.6815, 183.0868) radius 10
  circle A19 centre (-2.2876, 208.0868) radius 3 projected
  circle A20 centre (-2.2876, 208.0868) radius 10
  circle A21 centre (-83.0715, 260.0868) radius 10
  circle A22 centre (-8.0719, 243.0868) radius 10
  line L3 (-123.5719, -176.9752) -> (-123.5719, 478.248) projected
  line L4 (-92.5159, -211.9132) -> (-123.5719, -176.9752) projected
  line L5 (23.4281, -211.9132) -> (-92.5159, -211.9132) projected
  line L6 (-110.2837, 493.0975) -> (-75.5719, 531.8877) projected
  line L7 (-110.2837, 493.0975) -> (-110.2717, 493.0868) projected
  line L8 (-110.2717, 493.0868) -> (-110.2933, 493.0868) projected
  line L9 (-123.5719, 478.248) -> (-110.2933, 493.0868) projected
  point P0 (0, 0)
  dimension "d68" = 20
  dimension "d69" = 20
  dimension "d70" = 20
  dimension "d71" = 20
  dimension "d72" = 20
  dimension "d73" = 20
  dimension "d74" = 20
  constraints: 7 centre point, 7 coincident
  measures "d68" diameter of A12
  measures "d69" diameter of A14
  measures "d70" diameter of A16
  measures "d71" diameter of A18
  measures "d72" diameter of A20
  measures "d73" diameter of A21
  measures "d74" diameter of A22
extrude "Extrusion10" add sketch "Sketch10" along normal blind 15 contours A12 | A14 | A16 | A18 | A20 | A21 | A22
sketch "Sketch11" plane through (75, -187.1938, 138.5719) normal (1, 0, 0) x (0, 0, -1)
  circle A0 centre (55.5004, 287.2805) radius 10 projected
  circle A1 centre (55.5004, 447.2805) radius 10 projected
  circle A2 centre (100.8904, 370.2805) radius 10 projected
  circle A3 centre (136.2843, 245.2805) radius 10 projected
  circle A4 centre (130.5, 430.2805) radius 10 projected
  circle A5 centre (136.2843, 395.2805) radius 10 projected
  circle A6 centre (100.8904, 210.2805) radius 10 projected
  circle A7 centre (55.5, 105.2805) radius 9.5792 projected
  circle A8 centre (55.5, 535.2805) radius 15.3296 projected
  circle A9 centre (130.5, 105.2805) radius 11.2282 projected
  line L0 (63, 719.0815) -> (63, 746.0743) projected
  line L1 (28.2882, 680.2913) -> (63, 719.0815) projected
  line L2 (28.2882, 680.2913) -> (28.3002, 680.2805) projected
  line L3 (28.3002, 680.2805) -> (28.2786, 680.2805) projected
  line L4 (15, 665.4417) -> (28.2786, 680.2805) projected
  line L5 (15, 10.2186) -> (15, 665.4417) projected
  line L6 (46.056, -24.7195) -> (15, 10.2186) projected
  line L7 (162, -24.7195) -> (46.056, -24.7195) projected
  line L8 (162, -24.7195) -> (162, 409.5268) projected
  line L9 (162, 409.5268) -> (63, 746.0743) projected
  circle A10 centre (100.8904, 530.2805) radius 7.0135 projected
  line L10 (162, -24.7195) -> (162, -42.7195) projected
  line L11 (46.056, -24.7195) -> (162, -24.7195) projected
  line L12 (15, 10.2186) -> (46.056, -24.7195) projected
  line L13 (15, 665.4417) -> (15, 10.2186) projected
  line L14 (63, 719.0815) -> (15, 665.4417) projected
  line L15 (63, 746.0743) -> (63, 719.0815) projected
  line L16 (0, 675.6721) -> (63, 746.0743) projected
  line L17 (0, 0) -> (0, 675.6721) projected
  line L18 (37.9728, -42.7195) -> (0, 0) projected
  line L19 (162, -42.7195) -> (37.9728, -42.7195) projected
  line L20 (63, 746.0743) -> (63, 741.0743)
  line L21 (63, 719.0815) -> (63, 746.0743) projected
  line L22 (63, 741.0743) -> (15, 665.4417)
  point P0 (138.5719, 187.1938)
  dimension "d77" = 5
  constraints: 4 end point, 1 point on line
  measures "d77" distance of L15.start L20.end
extrude "Extrusion11" cut sketch "Sketch11" against normal up to surface (75 mm away) contours L1 L14 L4 L22 L0
sketch "Sketch12" plane through (0, -187.1938, 134.5719) normal (0, 0, 1) x (1, 0, 0)
  line L0 (10, 16) -> (10, 659.6721) projected
  line L1 (65, 16) -> (10, 16) projected
  line L2 (65, 659.6721) -> (65, 16) projected
  line L3 (10, 659.6721) -> (65, 659.6721) projected
  point P0 (0, 187.1938)
extrude "Extrusion12" add sketch "Sketch12" along normal up to surface (4 mm away)
ref_plane "Work Plane1" through (0, 558.8805, 75.5719) normal (0, -1, 0) x (1, 0, 0)
sketch "Sketch13" plane through (0, 558.8805, 75.5719) normal (0, -1, 0) x (1, 0, 0)
  line L0 (75, 63) -> (75, 0) projected
  line L1 (0, 0) -> (75, 0) projected
  line L2 (0, 63) -> (0, 0) projected
  line L3 (0, 63) -> (75, 63) projected
  line L4 (0, 48) -> (75, 48) projected
  line L5 (0, 48) -> (75, 48) projected
  line L6 (0, 48) -> (75, 48) projected
  line L7 (75, 48) -> (47, 48)
  line L8 (47, 48) -> (47, 35.3425)
  line L9 (47, 35.3425) -> (75, 35.3425)
  line L10 (75, 35.3425) -> (75, 48)
  line L11 (75, 48) -> (47, 48)
  line L12 (47, 48) -> (47, -4.7214)
  line L13 (47, -4.7214) -> (75, -4.7214)
  line L14 (75, -4.7214) -> (75, 48)
  line L15 (75, 25.0272) -> (75, 63) projected
  line L16 (47, 48) -> (75, 48)
  line L17 (75, 48) -> (75, 54)
  line L18 (75, 54) -> (47, 54)
  line L19 (47, 54) -> (47, 48)
  point P0 (0, -75.5719)
  dimension "d83" = 28
  dimension "d84" = 6
  constraints: 24 end point, 6 parallel, 3 horizontal, 3 perpendicular, 2 point on line
  measures "d83" distance of L9.end L8.end
  measures "d84" distance of L17.end L16.end
extrude "Extrusion13" cut sketch "Sketch13" along normal up to surface contours L0 L4 L19 L18 | L0 L9 L8 L4 | L0 L1 L12 L9 | L1 L14 L13 L12 surface through (0, -211.9132, 92.5159) normal (0, 0.6643638, -0.7474093)
sketch "Sketch14" plane through (75, -229.9132, -23.4281) normal (1, 0, 0) x (0, 0, -1)
  line L0 (-99.944, 0) -> (-153, 59.688) projected
  line L1 (-153, 59.688) -> (-153, 728.449) projected
  line L2 (-162, 718.3915) -> (-153, 728.449) projected
  line L3 (-162, 42.7195) -> (-162, 718.3915) projected
  line L4 (-124.0272, 0) -> (-162, 42.7195) projected
  line L5 (-99.944, 0) -> (-124.0272, 0) projected
  line L6 (-94.2786, 18) -> (-94.2786, 0) projected
  line L7 (0, 0) -> (-94.2786, 0) projected
  line L8 (0, 18) -> (0, 0) projected
  line L9 (-94.2786, 18) -> (0, 18) projected
  line L10 (-94.2786, 0) -> (-99.944, 0) projected
  line L11 (-94.2786, 18) -> (-94.2786, 0) projected
  line L12 (-115.944, 18) -> (-94.2786, 18) projected
  line L13 (-115.944, 18) -> (-99.944, 0) projected
  point P0 (-23.4281, 229.9132)
  point P1 (-94.2786, 18)
  point P2 (-115.944, 18)
extrude "Extrusion14" add sketch "Sketch14" against normal up to surface (28 mm away) contours L0 L12 L6 L10
sketch "Sketch15" plane through (0, -187.1938, 138.5719) normal (0, 0, 1) x (1, 0, 0)
  line L0 (75, 0) -> (75, 675.6721) projected
  line L1 (0, 675.6721) -> (75, 675.6721) projected
  line L2 (0, 0) -> (0, 675.6721) projected
  line L3 (0, 0) -> (75, 0) projected
  line L4 (47, 685.7295) -> (47, 16.9686) projected
  line L5 (0, 675.6721) -> (75, 675.6721) projected
  line L6 (47, 675.6721) -> (75, 675.6721)
  line L7 (61, 675.6721) -> (61, 645.6721)
  circle A0 centre (61, 645.6721) radius 4
  circle A1 centre (61, 645.6721) radius 2.1
  point P0 (0, 187.1938)
  dimension "d89" = 30
  dimension "d90" = 8
  dimension "d91" = 4.2
  constraints: 4 end point, 2 centre point, 2 coincident, 2 point on line, 1 collinear, 1 midpoint, 1 vertical
  measures "d89" distance of L7.start L7.end
  measures "d90" diameter of A0
  measures "d91" diameter of A1
extrude "Extrusion15" cut sketch "Sketch15" against normal blind 6 contours A0 | A1
extrude "Extrusion16" cut sketch "Sketch15" against normal through all contours A1
sketch "Sketch16" plane through (0, -187.1938, 138.5719) normal (0, 0, 1) x (1, 0, 0)
  line L0 (47, 685.7295) -> (47, 16.9686) projected
  circle A0 centre (61, 645.6721) radius 4 projected
  line L1 (75, 0) -> (75, 675.6721) projected
  line L2 (0, 675.6721) -> (75, 675.6721) projected
  line L3 (0, 0) -> (0, 675.6721) projected
  line L4 (0, 0) -> (75, 0) projected
  line L5 (75, 685.7295) -> (47, 685.7295) projected
  line L6 (47, 685.7295) -> (47, 746.0743) projected
  line L7 (0, 746.0743) -> (47, 746.0743) projected
  line L8 (0, 675.6721) -> (0, 746.0743) projected
  line L9 (0, 675.6721) -> (75, 675.6721) projected
  line L10 (75, 675.6721) -> (75, 685.7295) projected
  circle A1 centre (61, 645.6721) radius 2.1 projected
  line L11 (61, 645.6721) -> (61, 668.1821)
  line L12 (61, 668.1821) -> (61, 603.6928)
  circle A2 centre (61, 668.1821) radius 4
  circle A3 centre (61, 668.1821) radius 2.1
  point P0 (0, 187.1938)
  constraints: 4 end point, 2 centre point, 2 coincident, 1 point on line, 1 vertical
extrude "Extrusion17" cut sketch "Sketch16" against normal up to surface (6 mm away) contours A2 | A3
extrude "Extrusion18" cut sketch "Sketch16" against normal through all contours A3
sketch "Sketch17" plane through (0, -187.1938, 138.5719) normal (0, 0, 1) x (1, 0, 0)
  circle A0 centre (61, 668.1821) radius 4 projected
  circle A1 centre (61, 645.6721) radius 4 projected
  line L0 (75, 0) -> (75, 675.6721) projected
  line L1 (0, 675.6721) -> (75, 675.6721) projected
  line L2 (0, 0) -> (0, 675.6721) projected
  line L3 (0, 0) -> (75, 0) projected
  circle A2 centre (61, 645.6721) radius 4 projected
  line L4 (61, 645.6721) -> (61, 668.1821) construction
  line L5 (65, 645.6721) -> (65, 668.1821)
  line L6 (57, 668.1821) -> (57, 645.6721)
  arc A3 (57, 645.6721) -> (65, 645.6721) centre (61, 645.6721) ccw
  arc A4 (65, 668.1821) -> (57, 668.1821) centre (61, 668.1821) ccw
  point P0 (0, 187.1938)
  point P1 (61, 656.9271)
  constraints: 8 end point, 4 point on circle, 4 tangent, 2 centre point, 1 midpoint, 1 parallel, 1 vertical
extrude "Extrusion19" cut sketch "Sketch17" against normal up to surface (6 mm away) contours L5 A1 L6 A0
fillet "Fillet1" radius 0.5 2 edges at (23.5, 558.8805, 75.5719) (23.5, 553.8805, 75.5719)
sketch "Sketch18" plane through (0, -187.1938, 138.5719) normal (0, 0, 1) x (1, 0, 0)
  line L0 (75, 0) -> (75, 675.6721) projected
  line L1 (0, 675.6721) -> (75, 675.6721) projected
  line L2 (0, 0) -> (0, 675.6721) projected
  line L3 (0, 0) -> (75, 0) projected
  line L4 (65, 668.1821) -> (65, 645.6721) projected
  arc A0 (57, 645.6721) -> (65, 645.6721) centre (61, 645.6721) ccw projected
  line L5 (57, 645.6721) -> (57, 668.1821) projected
  arc A1 (65, 668.1821) -> (57, 668.1821) centre (61, 668.1821) ccw projected
  circle A2 centre (61, 645.6721) radius 2.1 projected
  arc A3 (65, 668.1821) -> (57, 668.1821) centre (61, 668.1821) ccw projected
  line L6 (57, 645.6721) -> (57, 668.1821) projected
  arc A4 (57, 645.6721) -> (65, 645.6721) centre (61, 645.6721) ccw projected
  line L7 (65, 668.1821) -> (65, 645.6721) projected
  circle A5 centre (61, 645.6721) radius 2.1 projected
  line L8 (61, 645.6721) -> (67, 645.6721)
  line L9 (61, 645.6721) -> (57, 645.6721)
  arc A6 (57, 645.6721) -> (65, 645.6721) centre (61, 645.6721) ccw projected
  line L10 (67, 645.6721) -> (57, 645.6721) construction
  line L11 (67, 643.5721) -> (57, 643.5721)
  line L12 (57, 647.7721) -> (67, 647.7721)
  arc A7 (67, 643.5721) -> (67, 647.7721) centre (67, 645.6721) ccw
  arc A8 (57, 647.7721) -> (57, 643.5721) centre (57, 645.6721) ccw
  circle A9 centre (61, 668.1821) radius 2.1 projected
  line L13 (61, 668.1821) -> (57, 668.1821)
  line L14 (57, 645.6721) -> (57, 668.1821) projected
  line L15 (61, 668.1821) -> (67, 668.1821)
  line L16 (57, 668.1821) -> (67, 668.1821) construction
  line L17 (57, 666.0821) -> (67, 666.0821)
  line L18 (67, 670.2821) -> (57, 670.2821)
  arc A10 (57, 670.2821) -> (57, 666.0821) centre (57, 668.1821) ccw
  arc A11 (67, 666.0821) -> (67, 670.2821) centre (67, 668.1821) ccw
  line L19 (67, 645.6721) -> (57, 645.6721) construction
  line L20 (67, 649.6721) -> (57, 649.6721)
  line L21 (57, 641.6721) -> (67, 641.6721)
  arc A12 (67, 641.6721) -> (67, 649.6721) centre (67, 645.6721) ccw
  arc A13 (57, 649.6721) -> (57, 641.6721) centre (57, 645.6721) ccw
  line L22 (67, 668.1821) -> (57, 668.1821) construction
  line L23 (67, 672.1821) -> (57, 672.1821)
  line L24 (57, 664.1821) -> (67, 664.1821)
  arc A14 (67, 664.1821) -> (67, 672.1821) centre (67, 668.1821) ccw
  arc A15 (57, 672.1821) -> (57, 664.1821) centre (57, 668.1821) ccw
  point P0 (0, 187.1938)
  point P1 (62, 645.6721)
  point P2 (62, 668.1821)
  point P3 (62, 645.6721)
  point P4 (62, 668.1821)
  point P5 (65, 664.1821)
  point P6 (65, 649.6721)
  point P7 (61, 672.1821)
  point P8 (61, 641.6721)
  point P9 (61, 643.5721)
  point P10 (61, 647.7721)
  dimension "d103" = 6
  dimension "d104" = 4
  dimension "d105" = 6
  dimension "d106" = 8
  dimension "d107" = 8
  constraints: 40 end point, 16 point on circle, 16 tangent, 8 centre point, 5 parallel, 4 horizontal, 4 midpoint, 2 point on line, 1 perpendicular
  measures "d103" distance of L8.start L8.end
  measures "d104" distance of L8.start L6.start
  measures "d105" distance of L13.start L15.end
  measures "d106" diameter of A13
  measures "d107" diameter of A15
extrude "Extrusion20" add sketch "Sketch18" against normal up to surface (6 mm away) contours L4 L20 L5 L24
extrude "Extrusion21" cut sketch "Sketch18" against normal up to surface (6 mm away) contours A1 L18 A11 L17 L4 | L17 A11 L18 A1 L23 A14 L24 L4 | A1 L18 A10 L5 A15 L23 | L20 A12 L21 A0 L11 A7 L12 L4 | A10 L18 A1 L5 | L12 A7 L11 A0 L4 | L5 A8 L11 A0 L21 A13 | L5 A0 L11 A8
extrude "Extrusion22" cut sketch "Sketch18" against normal through all contours A1 L18 A11 L17 L4 | L15 A9 L18 A1 | L4 L17 A9 L15 | L15 L13 A9 | A9 L13 L15 | L17 L5 L13 A9 | A9 L13 A1 L18 | A10 L18 A1 L5 | L12 A7 L11 A0 L4 | L4 L8 A2 L12 | A0 L11 A2 L8 | A2 L9 L5 L12 | L5 A0 L11 A8 | A2 L11 A0 L9
sketch "Sketch19" plane through (75, 498.5358, 129.5719) normal (0, 0, -1) x (-1, 0, 0)
  line L0 (8, -15.4474) -> (18, -15.4474) projected
  arc A0 (18, -19.6474) -> (18, -15.4474) centre (18, -17.5474) ccw projected
  line L1 (18, -19.6474) -> (8, -19.6474) projected
  arc A1 (8, -15.4474) -> (8, -19.6474) centre (8, -17.5474) ccw projected
  line L2 (8, -37.9575) -> (18, -37.9575) projected
  arc A2 (18, -42.1575) -> (18, -37.9575) centre (18, -40.0575) ccw projected
  line L3 (18, -42.1575) -> (8, -42.1575) projected
  arc A3 (8, -37.9575) -> (8, -42.1575) centre (8, -40.0575) ccw projected
  line L4 (0, 0) -> (28, 0) projected
  line L5 (0, -668.7609) -> (0, 0) projected
  line L6 (0, -668.7609) -> (28, -668.7609) projected
  line L7 (28, 0) -> (28, -668.7609) projected
  line L8 (0, -710.449) -> (0, -668.7609) projected
  line L9 (28, -668.7609) -> (0, -668.7609)
  line L10 (0, -668.7609) -> (0, -689.605)
  line L11 (0, -689.605) -> (28, -689.605)
  line L12 (28, -689.605) -> (28, -668.7609)
  point P0 (75, -498.5358)
  constraints: 8 end point, 2 parallel, 1 horizontal, 1 midpoint, 1 perpendicular
extrude "Extrusion23" add sketch "Sketch19" along normal blind 2
sketch "Sketch20" plane through (47, -176.9752, 123.5719) normal (1, 0, 0) x (0, 0, -1)
  line L0 (-6, 675.5109) -> (-4, 675.5109) projected
  line L1 (-4, 675.5109) -> (-4, 4.5) projected
  line L2 (-4, 4.5) -> (0, 0) projected
  line L3 (0, 655.2231) -> (0, 0) projected
  line L4 (47.9222, 730.733) -> (0, 655.2231) projected
  arc A0 (47.9222, 730.733) -> (48, 731.0009) centre (47.5, 731.0009) ccw projected
  line L5 (48, 734.5471) -> (48, 731.0009) projected
  arc A1 (48, 734.5471) -> (47.1274, 734.8805) centre (47.5, 734.5471) ccw projected
  line L6 (-6, 675.5109) -> (47.1274, 734.8805) projected
  line L7 (-15, 665.4535) -> (-6, 675.5109) projected
  line L8 (-15, -10.2186) -> (-15, 665.4535) projected
  line L9 (22.9728, -52.938) -> (-15, -10.2186) projected
  line L10 (147, -52.938) -> (22.9728, -52.938) projected
  line L11 (147, -34.938) -> (147, -52.938) projected
  line L12 (31.056, -34.938) -> (147, -34.938) projected
  line L13 (31.056, -34.938) -> (-4, 4.5) projected
  line L14 (-4, 675.5109) -> (-4, 4.5) projected
  line L15 (-6, 675.5109) -> (-4, 675.5109) projected
  line L16 (-4, 675.5109) -> (-4, 677.7459)
  point P0 (123.5719, 176.9752)
  constraints: 2 end point, 1 point on line, 1 vertical
extrude "Extrusion24" add sketch "Sketch20" along normal up to surface (28 mm away) contours L6 L16 L0
sketch "Sketch21" plane through (0, -187.1938, 132.5719) normal (0, 0, 1) x (1, 0, 0)
  line L0 (57, 647.7721) -> (67, 647.7721) projected
  arc A0 (67, 643.5721) -> (67, 647.7721) centre (67, 645.6721) ccw projected
  line L1 (67, 643.5721) -> (57, 643.5721) projected
  arc A1 (57, 647.7721) -> (57, 643.5721) centre (57, 645.6721) ccw projected
  line L2 (67, 649.6721) -> (57, 649.6721) projected
  arc A2 (57, 649.6721) -> (57, 641.6721) centre (57, 645.6721) ccw projected
  line L3 (67, 641.6721) -> (57, 641.6721) projected
  arc A3 (67, 641.6721) -> (67, 649.6721) centre (67, 645.6721) ccw projected
  line L4 (67, 666.0821) -> (57, 666.0821) projected
  line L5 (67, 666.0821) -> (57, 666.0821) projected
  arc A4 (57, 670.2821) -> (57, 666.0821) centre (57, 668.1821) ccw projected
  line L6 (57, 670.2821) -> (67, 670.2821) projected
  arc A5 (67, 666.0821) -> (67, 670.2821) centre (67, 668.1821) ccw projected
  line L7 (57, 664.1821) -> (67, 664.1821) projected
  arc A6 (67, 664.1821) -> (67, 672.1821) centre (67, 668.1821) ccw projected
  line L8 (57, 672.1821) -> (67, 672.1821) projected
  arc A7 (57, 672.1821) -> (57, 664.1821) centre (57, 668.1821) ccw projected
  point P0 (0, 187.1938)
extrude "Extrusion25" cut sketch "Sketch21" against normal blind 2
sketch "Sketch22" plane through (0, 0, 0) normal (1, 0, 0) x (0, 0, -1)
  circle A0 centre (-83.0719, -81.9132) radius 9.5792 projected
  circle A1 centre (-8.0719, -81.9132) radius 11.2282 projected
  circle A2 centre (-37.6815, 343.0868) radius 7.0135 projected
  circle A3 centre (-83.0719, 348.0868) radius 15.3296 projected
  circle A4 centre (-8.0719, 243.0868) radius 10 projected
  circle A5 centre (-83.0715, 260.0868) radius 10 projected
  circle A6 centre (-2.2876, 58.0868) radius 10 projected
  circle A7 centre (-83.0715, 100.0868) radius 10 projected
  point P0 (0, 0)
extrude "Extrusion26" cut sketch "Sketch22" along normal through all